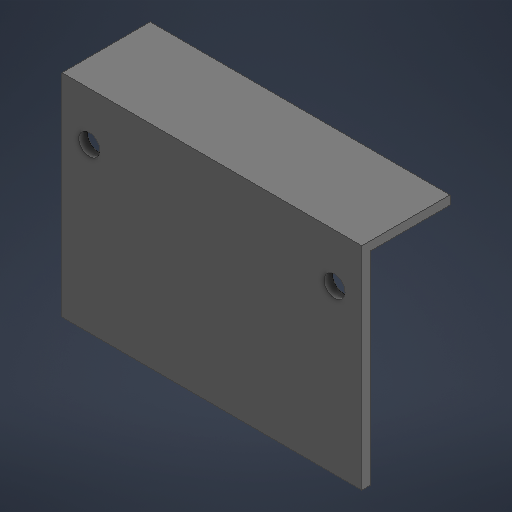
# Autodesk Inventor part: MainsCover
Saved by Autodesk Inventor 2026.2 (Build 302298010, 298A)
## iProperties
Created: 2026-08-03
Part Number: MainsCover
Material: Generic
Document SubType Name: Modeling
Designer: sonata
Density: 1 g/cm^3
Appearance: Default
Author: sonata
Autodesk Inventor part; units mm, degrees
ref_plane "YZ Plane" through (0, 0, 0) normal (1, 0, 0) x (0, 1, 0)
ref_plane "XZ Plane" through (0, 0, 0) normal (0, 1, 0) x (-1, 0, 0)
ref_plane "XY Plane" through (0, 0, 0) normal (0, 0, 1) x (1, 0, 0)
sketch "Sketch1" plane through (0, 0, 0) normal (0, 0, 1) x (1, 0, 0)
  line L0 (0, 0) -> (68, 0)
  line L1 (68, 0) -> (68, 48)
  line L2 (68, 48) -> (0, 48)
  line L3 (0, 48) -> (0, 0)
  dimension "d0" = 68
  dimension "d1" = 48
  constraints: 8 end point, 2 parallel, 1 horizontal, 1 perpendicular
  measures "d0" distance of L1.end L2.end
  measures "d1" distance of L0.end L1.end
extrude "Extrusion1" add sketch "Sketch1" along normal blind 2
sketch "Sketch2" plane through (0, 0, 2) normal (0, 0, 1) x (1, 0, 0)
  circle A0 centre (6.2, 37) radius 2.4
  circle A1 centre (61.8, 37) radius 2.4
  line L0 (0, 0) -> (68, 0) projected
  line L1 (34, 0) -> (34, 48) construction
  line L2 (68, 48) -> (0, 48) projected
  dimension "d4" = 4.8
  dimension "d5" = 4.8
  dimension "d6" = 55.6
  dimension "d7" = 27.8
  dimension "d8" = 37
  constraints: 2 centre point, 2 end point, 2 midpoint, 1 horizontal alignment
  measures "d4" diameter of A0
  measures "d5" diameter of A1
  measures "d6" distance of A1.centre A0.centre
  measures "d7" distance from line of L1 A0.centre
  measures "d8" distance from line of A0.centre L0
extrude "Extrusion2" cut sketch "Sketch2" against normal blind 2
sketch "Sketch3" plane through (0, 0, 0) normal (0, 0, -1) x (-1, 0, 0)
  line L0 (-68, 48) -> (0, 48)
  line L1 (0, 48) -> (0, 46)
  line L2 (0, 46) -> (-68, 46)
  line L3 (-68, 46) -> (-68, 48)
  line L4 (0, 0) -> (0, 2)
  line L5 (-68, 2) -> (-68, 0)
  dimension "d11" = 2
  constraints: 12 end point, 3 parallel, 1 horizontal, 1 perpendicular
  measures "d11" distance between parallel lines of L0 L2
extrude "Extrusion3" add sketch "Sketch3" along normal blind 18
body "Solid1"
